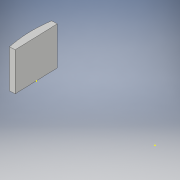
# Autodesk Inventor part: Speaker Mount 1
Saved by Autodesk Inventor 2019 (Build 230136000, 136)
## iProperties
Created: 2019-06-28
Part Number: Speaker Mount 1
Material: Generic
Document SubType Name: Modeling
Designer: Baldwin
Density: 1 g/cm^3
Appearance: Default
Author: Baldwin
Autodesk Inventor part; units mm, degrees
ref_plane "YZ Plane" through (0, 0, 0) normal (1, 0, 0) x (0, 1, 0)
ref_plane "XZ Plane" through (0, 0, 0) normal (0, 1, 0) x (-1, 0, 0)
sketch "Sketch1" plane through (0, 0, 0) normal (0, 1, 0) x (-1, 0, 0)
  point P0 (0, 0)
sketch "Sketch2" plane through (0, 0, 0) normal (0, 1, 0) x (-1, 0, 0)
  circle A0 centre (0, 0) radius 225
  dimension "d0" = 450
  constraints: 1 centre point, 1 coincident
  measures "d0" diameter of A0
extrude "Extrusion1" add sketch "Sketch2" along normal blind 70
sketch "Sketch3" plane through (0, 70, 0) normal (0, 1, 0) x (1, 0, 0)
  circle A0 centre (0, 0) radius 225 projected
  line L0 (-222.5878, 32.8586) -> (-220.015, -47.1001)
  dimension "d3" = 80
  constraints: 2 end point, 2 point on circle
  measures "d3" distance of L0.start L0.end
split body "Split1" sketch "Sketch3" result one side removed curves L0 removed pieces at (-39.9451, 0.5, -49.4831)
sketch "Sketch4" plane through (-220.015, 0, 47.1001) normal (0.9994827, 0, -0.03216) x (-0.03216, 0, -0.9994827)
  line L0 (80, 70) -> (0, 70) projected
  line L1 (0, 70) -> (80, 70)
  line L2 (80, 70) -> (80, 0)
  line L3 (80, 0) -> (0, 0)
  line L4 (0, 0) -> (0, 70)
  point P0 (40, 0)
  constraints: 8 end point, 2 parallel, 1 horizontal, 1 perpendicular
extrude "Extrusion2" add sketch "Sketch4" along normal blind 10
sketch "Sketch5" plane through (-210.0201, 0, 46.7785) normal (0.9994827, 0, -0.03216) x (-0.03216, 0, -0.9994827)
  point P0 (40, 0)
ref_plane "Work Plane1" through (-224.8836, 0, 7.236) normal (0.9994827, 0, -0.03216) x (0, 1, 0)
body "Solid1"
